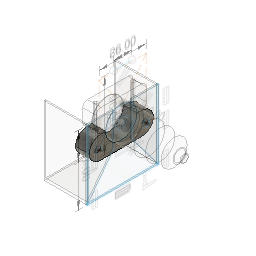
drill-clamp-43mm (Autodesk Fusion 360 design; units mm, degrees)
Autodesk Fusion 360 part; units mm, degrees
sketch "Sketch1" plane through (0, 0, 0) normal (1, 0, 0) x (0, 1, 0) in component "frame"
  line L0 (-50, 0) -> (50, 0)
  line L1 (50, 0) -> (50, -97)
  line L2 (50, -97) -> (-50, -97)
  line L3 (-50, -97) -> (-50, 0)
  line L4 (-13, -48) -> (-13, 0)
  line L5 (-13, 48) -> (13, 48)
  line L6 (13, 0) -> (13, -48)
  line L7 (-13, -48) -> (-50, -97)
  line L8 (13, -48) -> (50, -97)
  line L9 (-50, 0) -> (50, 0) construction
  line L10 (50, 0) -> (50, -39) construction
  line L11 (50, -39) -> (-50, -39) construction
  line L12 (-50, -39) -> (-50, 0) construction
  line L13 (33, -46.0191) -> (-33, -46.0191) construction
  line L14 (-33, -46.0191) -> (-33, 46.0191) construction
  line L15 (-33, 46.0191) -> (33, 46.0191) construction
  line L16 (33, 46.0191) -> (33, -46.0191) construction
  line L17 (33, -46.0191) -> (-33, 46.0191) construction
  line L18 (-33, -46.0191) -> (33, 46.0191) construction
  circle A0 centre (-33, -39) radius 4.5
  circle A1 centre (33, -39) radius 4.5
  line L19 (-50, -97) -> (50, -97)
  line L20 (50, -97) -> (50, -95)
  line L21 (50, -95) -> (-50, -95)
  line L22 (-50, -95) -> (-50, -97)
  line L23 (50, 0) -> (48, 0)
  line L24 (48, 0) -> (48, -97)
  line L25 (48, -97) -> (50, -97)
  line L26 (50, -97) -> (50, 0)
  line L27 (-50, 0) -> (-48, 0)
  line L28 (-48, 0) -> (-48, -97)
  line L29 (-48, -97) -> (-50, -97)
  line L30 (-50, -97) -> (-50, 0)
  dimension "d1" = 97
  dimension "d2" = 26
  dimension "d3" = 96
  dimension "d4" = 39
  dimension "d5" = 66
  dimension "d6" = 9
  dimension "d7" = 9
  dimension "d10" = 2
  dimension "d11" = 2
  constraint horizontal L0
  constraint vertical L1
  constraint horizontal L2
  constraint vertical L3
  constraint parallel L4 L6
  constraint coincident L0 L4.end
  constraint coincident L0 L6.start
  constraint horizontal L9
  constraint vertical L10
  constraint horizontal L11
  constraint vertical L12
  constraint horizontal L13
  constraint perpendicular L13 L14
  constraint parallel L13 L15
  constraint parallel L14 L16
  constraint coincident L17 origin
  constraint coincident L18 origin
  constraint coincident L14 A0.centre
  constraint coincident L11 A0.centre
  constraint coincident L16 A1.centre
  constraint coincident L11 A1.centre
  constraint horizontal L19
  constraint vertical L20
  constraint horizontal L21
  constraint vertical L22
  constraint coincident L1 L20.end
  constraint horizontal L23
  constraint vertical L24
  constraint horizontal L25
  constraint vertical L26
  constraint horizontal L27
  constraint vertical L28
  constraint horizontal L29
  constraint vertical L30
  measures "d1" distance of L0.start L2.end
  measures "d2" distance of L5.start L5.end
  measures "d3" distance of L4.start L5.start
  measures "d4" distance of L0.start L11.end
  measures "d5" distance of L14.end L15.end
  measures "d6" diameter of A0
  measures "d7" diameter of A1
  measures "d10" distance of L0.end L23.end
  measures "d11" distance of L0.start L27.end
extrude "Extrude2" add sketch "Sketch1" against normal blind 60 contours L0 L3 L7 L21 L27 L28 L30 | L3 L7 L21 L22 L30 | L7 L21 L28 | L2 L7 L19 L21 L28 L29 | L2 L19 L21 L24 L28 | L0 L1 L8 L21 L23 L24 L26 | L8 L21 L24 | L2 L8 L19 L21 L24 L25 | L1 L8 L20 L21 L26 makes body 1 in component "frame"
extrude "Extrude1" add sketch "Sketch1" against normal blind 2 separate body contours L0 L3 L7 L21 L27 L28 L30 | L0 L4 L7 L28 | L3 L7 L21 L22 L30 | L0 L6 L8 L24 | L0 L1 L8 L21 L23 L24 L26 | L1 L8 L20 L21 L26 makes body 2 at (0, -31.8879, -11.5042) makes body 3 at (0, 31.8879, -11.5042) in component "frame"
sketch "Sketch1 (2)" plane through (-2, 0, 0) normal (-1, 0, 0) x (0, -1, 0) in component "drill-bosh"
  circle A0 centre (0, -22) radius 21.5
  circle A1 centre (0, -22) radius 7
  dimension "d14" = 43
  dimension "d17" = 14
  constraint concentric A0 A1
  measures "d14" diameter of A0
  measures "d17" diameter of A1
extrude "Extrude2'" add sketch "Sketch1 (2)" against normal blind 7 separate body contours A1 makes body 4 in component "drill-bosh"
extrude "Extrude1'" add sketch "Sketch1 (2)" along normal blind 20 separate body contours A0 | A1 makes body 5 in component "drill-bosh"
sketch "Sketch3" plane through (5, 0, 0) normal (1, 0, 0) x (0, 1, 0) in component "drill-bosh"
  circle A0 centre (0, -22) radius 7
  circle A1 centre (0, -22) radius 21.5
  dimension "d20" = 43
  constraint concentric A0 A1
  measures "d20" diameter of A1
extrude "Extrude3" add sketch "Sketch3" along normal blind 40 contours A0 | A1 bodies 4 in component "drill-bosh"
sketch "Sketch4" plane through (45, 0, 0) normal (1, 0, 0) x (0, 1, 0) in component "drill-bosh"
  circle A0 centre (0, -22) radius 21.5
extrude "Extrude4" add sketch "Sketch4" along normal blind 35 draft -7 bodies 4 in component "drill-bosh"
sketch "Sketch5" plane through (80, 0, 0) normal (1, 0, 0) x (0, 1, 0) in component "drill-bosh"
  circle A0 centre (0, -22) radius 17.2025
  circle A1 centre (0, -22) radius 7.8103
  constraint concentric A0 A1
extrude "Extrude5" add sketch "Sketch5" along normal blind 7 draft -18 contours A1 bodies 4 in component "drill-bosh"
fillet "Fillet1" radius 9 1 edges at (80, -16.0384, -15.7793) on bodies 4 in component "drill-bosh"
fillet "Fillet2" radius 127 1 edges at (45, -20.045, -29.7747) on bodies 4 in component "drill-bosh"
fillet "Fillet3" radius 3 1 edges at (5, -20.045, -29.7747) on bodies 4 in component "drill-bosh"
fillet "Fillet4" radius 1 1 edges at (87, -5.1612, -19.9982) on bodies 4 in component "drill-bosh"
sketch "Sketch3 (2)" plane through (0, 0, 0) normal (1, 0, 0) x (0, 1, 0) in component "clamp-top"
  arc A0 (21.9945, -21.5073) -> (-21.9942, -21.495) centre (0, -22) ccw
  line L0 (-21.9942, -21.495) -> (-35, -21.495)
  line L1 (21.9945, -21.5073) -> (35, -21.5073)
  line L2 (-35, -21.495) -> (-35, 10)
  line L3 (-35, 10) -> (35, 10)
  line L4 (35, 10) -> (35, -21.5073)
  dimension "d35" = 22
  constraint horizontal L0
  constraint horizontal L1
  constraint perpendicular L2 L3
  measures "d35" radius of A0
extrude "Extrude1''" add sketch "Sketch3 (2)" against normal blind 19 separate body makes body 6 in component "clamp-top"
sketch "Sketch1 (3)" plane through (-2, 0, 0) normal (-1, 0, 0) x (0, -1, 0) in component "clamp-bottom"
  arc A0 (-22, -22.5) -> (22, -22.5) centre (0, -22) ccw
  line L0 (22, -22.5) -> (45, -22.5)
  line L1 (45, -22.5) -> (45, -53.924)
  line L2 (45, -53.924) -> (-45, -53.924)
  line L3 (-22, -22.5) -> (-45, -22.5)
  line L4 (-45, -22.5) -> (-45, -53.924)
  circle A1 centre (-33, -39) radius 3.5
  circle A2 centre (33, -39) radius 3.5
  dimension "d39" = 7
  dimension "d40" = 7
  constraint horizontal L0
  constraint perpendicular L0 L1
  constraint perpendicular L1 L2
  constraint horizontal L3
  constraint perpendicular L2 L4
  measures "d39" diameter of A1
  measures "d40" diameter of A2
extrude "Extrude1'''" add sketch "Sketch1 (3)" along normal up to surface (19 mm away) separate body makes body 7 in component "clamp-bottom"
sketch "Sketch4 (2)" plane through (0, 0, -53.924) normal (0, 0, -1) x (1, 0, 0) in component "clamp-bottom"
  line L0 (-21, 45) -> (-21, -45)
  line L1 (-21, -45) -> (-2, -45)
  line L2 (-2, -45) -> (-2, 45)
  line L3 (-2, 45) -> (-21, 45)
  line L4 (-14.5, 26) -> (-12.26, 27.68)
  line L5 (-14.5, 26) -> (-12.26, 24.32)
  arc A0 (-12.26, 24.32) -> (-12.26, 27.68) centre (-11, 26) ccw
  line L6 (-14.5, -26) -> (-12.26, -24.32)
  line L7 (-14.5, -26) -> (-12.26, -27.68)
  arc A1 (-12.26, -27.68) -> (-12.26, -24.32) centre (-11, -26) ccw
  dimension "d51" = 4.2
  dimension "d52" = 4.2
  constraint tangent L4 A0
  constraint tangent L5 A0
  constraint tangent L6 A1
  constraint tangent L7 A1
  measures "d51" diameter of A0
  measures "d52" diameter of A1
extrude "Extrude2''" cut sketch "Sketch4 (2)" against normal blind 80 contours L4 L5 A0 | L6 L7 A1 sketch seen with x (1, 0, 0) y (0, 1, 0) z (0, 0, 1) at (2, 0, 0) bodies 6 in component "clamp-top"
extrude "Extrude2'''" cut sketch "Sketch4 (2)" against normal blind 80 contours L4 L5 A0 | L6 L7 A1 bodies 7 in component "clamp-bottom"
fillet "Fillet1'" radius 16 4 edges at (-11.5, 45, -22.5) (-11.5, 45, -53.924) (-11.5, -45, -22.5) (-11.5, -45, -53.924) on bodies 7 in component "clamp-bottom"
fillet "Fillet1''" radius 6.5 2 edges at (-9.5, -35, -21.495) (-9.5, 35, -21.5073) on bodies 6 in component "clamp-top"
fillet "Fillet2'" radius 6.5 2 edges at (-9.5, -35, 10) (-9.5, 35, 10) on bodies 6 in component "clamp-top"
component "clamp-top" placed x (1, 0, 0) y (0, 1, 0) z (0, 0, 1) at (-2, 0, 0)
component "frame" placed x (1, 0, 0) y (0, 1, 0) z (0, 0, 1) at (0, 0, 0)
component "drill-bosh" placed x (1, 0, 0) y (0, 1, 0) z (0, 0, 1) at (0, 0, 0)
component "clamp-bottom" placed x (1, 0, 0) y (0, 1, 0) z (0, 0, 1) at (0, 0, 0)
equation "d3 = ( 48 * 2 ) * 1 mm"
equation "d4 = 34.5 mm + 4.5 mm"
